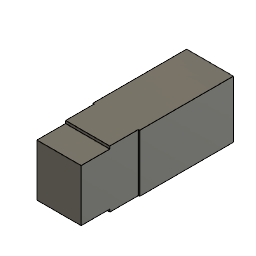
Mt1-2 (Autodesk Fusion 360 archive; units mm, degrees)
design "Esterno1"
part number: 2026-07-15-12-18-51-042
Autodesk Fusion 360 part; units mm, degrees
note: some values were not read from the file. Chosen so that the rebuilt part matches the saved one: which pieces of a blend or face edit are solid.
sketch "Schizzo1" plane through (0, 0, 0) normal (0, 1, 0) x (1, 0, 0)
sketch "Schizzo2" plane through (0, 0, 0) normal (0, 1, 0) x (1, 0, 0)
  line L0 (0, 0) -> (18, 0)
  line L1 (18, 0) -> (18, -36)
  line L2 (18, -36) -> (0, -36)
  line L3 (0, -36) -> (0, 0)
  line L4 (0, -36) -> (0.5, -36)
  line L5 (0.5, -36) -> (17.5, -36)
  line L6 (17.5, -36) -> (17.5, -47)
  line L7 (17.5, -47) -> (0.5, -47)
  line L8 (0.5, -47) -> (0.5, -36)
  dimension "d1" = 36
  dimension "d2" = 18
  dimension "d3" = 0.5
  dimension "d4" = 11
  dimension "d5" = 17
  constraint horizontal L0
  constraint vertical L1
  constraint horizontal L2
  constraint vertical L3
  constraint coincident L0.start L3.end
  constraint perpendicular L3 L4
  constraint horizontal L5
  constraint vertical L6
  constraint horizontal L7
  constraint vertical L8
  measures "d1" distance of L0.start L2.end
  measures "d2" distance of L1 L3
  measures "d3" distance of L2.end L4.end
  measures "d4" distance of L4.end L7.end
  measures "d5" distance of L6.end L7.end
extrude "Estrusione1" add sketch "Schizzo2" along normal blind 22
sketch "Schizzo3" plane through (0, 0, 47) normal (0, 0, 1) x (1, 0, 0)
  line L0 (0.5, 0) -> (17.5, 0)
  line L1 (17.5, 0) -> (17.5, 22)
  line L2 (17.5, 22) -> (0.5, 22)
  line L3 (0.5, 22) -> (0.5, 0)
  line L4 (0.5, 22) -> (17.5, 22)
  line L5 (0.5, 22) -> (0.5, 21)
  line L6 (0.5, 21) -> (17.5, 21)
  line L7 (17.5, 21) -> (17.5, 1)
  line L8 (17.5, 1) -> (0.5, 1)
  line L9 (0.5, 1) -> (0.5, 21)
  dimension "d8" = 20
  dimension "d9" = 17
  constraint coincident L2.end L3.start
  constraint coincident L1.end L2.start
  constraint coincident L3 L5.end
  constraint horizontal L6
  constraint vertical L7
  constraint horizontal L8
  constraint vertical L9
  measures "d8" distance of L5.end L8.end
  measures "d9" distance of L7.end L8.end
extrude "Estrusione2" add sketch "Schizzo3" along normal blind 11 contours L1 L3 L6 L7 L8 L9
sketch "Schizzo4" plane through (0, 0, 0) normal (0, 0, 1) x (1, 0, 0)
  line L0 (0, 0) -> (9, 0)
  line L1 (9, 0) -> (9, 6)
  line L2 (9, 6) -> (7, 6)
  line L3 (7, 6) -> (11, 6)
  line L4 (11, 6) -> (11, 11)
  line L5 (11, 11) -> (7, 11)
  line L6 (7, 11) -> (7, 6)
  dimension "d12" = 6
  constraint coincident L0.start origin
  constraint horizontal L0
  constraint perpendicular L0 L1
  constraint perpendicular L1 L2
  constraint horizontal L3
  constraint vertical L4
  constraint horizontal L5
  constraint vertical L6
  measures "d12" distance of L0.end L1.end
extrude "Estrusione3" add sketch "Schizzo4" against normal blind 5
sketch "Schizzo5" plane through (0, 0, 0) normal (-1, 0, 0) x (0, 0, 1)
  line L0 (0, 0) -> (36, 0)
  line L1 (36, 0) -> (36, 22)
  line L2 (36, 22) -> (0, 22)
  line L3 (0, 22) -> (0, 0)
  line L4 (0, 0) -> (0, 11)
  line L5 (0, 11) -> (9, 11)
  line L6 (9, 11) -> (11.5, 11)
  circle A0 centre (11.5, 11) radius 1.375
  dimension "d15" = 11
  dimension "d16" = 9
  dimension "d17" = 2.5
  dimension "d18" = 2.75
  constraint coincident L0.start L3.end
  constraint perpendicular L2 L4
  constraint perpendicular L4 L5
  constraint parallel L5 L6
  constraint coincident L6.end A0.centre
  measures "d15" distance of L0.start L4.end
  measures "d16" distance of L4.end L5.end
  measures "d17" distance of L5.end L6.end
  measures "d18" diameter of A0
extrude "Estrusione4" add sketch "Schizzo5" along normal blind 10 contours A0
move_face "Sposta faccia1" to x (-1, 0, 0) y (0, -0.939924, 0.341384) z (0, 0.341384, 0.939924) at (18.9949, 16.8905, -3.0643) 1 faces at (-3.3333, 11.0685, 12.8733)
